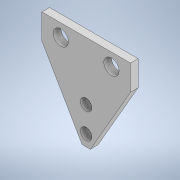
# Autodesk Inventor part: Load Cell Connector to Extrusion Bar
Saved by Autodesk Inventor 2022 (Build 260153000, 153)
## iProperties
Created: 2022-09-20
Part Number: Load Cell Connector to Extrusion Bar
Material: Generic
Document SubType Name: Modeling
Designer: Garrett Raker
Density: 1 g/cm^3
Appearance: Default
Author: Garrett Raker
Autodesk Inventor part; units mm, degrees
ref_plane "YZ Plane" through (0, 0, 0) normal (1, 0, 0) x (0, 1, 0)
ref_plane "XZ Plane" through (0, 0, 0) normal (0, 1, 0) x (-1, 0, 0)
ref_plane "XY Plane" through (0, 0, 0) normal (0, 0, 1) x (1, 0, 0)
sketch "Sketch1" plane through (0, 0, 0) normal (0, 0, 1) x (1, 0, 0)
  circle A0 centre (-10, 13.9812) radius 3
  circle A1 centre (10, 13.9812) radius 3
  circle A2 centre (0, -4.0188) radius 2.25
  circle A3 centre (0, -14.0188) radius 2.25
  line L0 (-1.6291, -18.508) -> (1.6291, -18.508)
  line L1 (-17.5, 8.9812) -> (-1.6291, -18.508)
  line L2 (-17.5, 8.9812) -> (17.1989, 8.9812) construction
  line L3 (17.5, 8.9812) -> (1.6291, -18.508)
  line L4 (17.5, 8.9812) -> (62.1106, 8.9812) construction
  line L5 (-17.5, 8.9812) -> (-17.5, 18.9812)
  line L6 (-17.5, 18.9812) -> (17.5, 18.9812)
  line L7 (17.5, 18.9812) -> (17.5, 8.9812)
  point P0 (0, -18.508)
  dimension "d1" = 4.5
  dimension "d2" = 10
  dimension "d3" = 6
  dimension "d4" = 10
  dimension "d5" = 60
  dimension "d10" = 35
  dimension "d11" = 17.5
  dimension "d13" = 3.2582
  dimension "d17" = 120
  dimension "d20" = 10
  dimension "d22" = 23
  dimension "d26" = 5
  constraints: 16 end point, 5 horizontal, 4 centre point, 2 equal radius, 1 horizontal alignment, 1 midpoint, 1 parallel, 1 perpendicular, 1 vertical, 1 vertical alignment
  measures "d1" diameter of A2
  measures "d2" distance of A2.centre A3.centre
  measures "d3" diameter of A0
  measures "d4" horizontal distance of A1.centre A2.centre
  measures "d5" angle of L1 L2
  measures "d10" distance between parallel lines of L7 L5
  measures "d11" distance from line of A2.centre L5
  measures "d13" distance of L0.start L0.end
  measures "d17" angle of L0 L3
  measures "d20" distance of L1.start L5.end
  measures "d22" distance from line of A2.centre L6
  measures "d26" distance from line of A0.centre L6
extrude "Extrusion1" add sketch "Sketch1" along normal blind 3
ref_plane "Work Plane4" through (-10, 13.9812, 0) normal (1, 0, 0) x (0, 0, -1)
ref_plane "Work Plane1" through (-13, 13.9812, 0) normal (-1, 0, 0) x (0, 0, 1)
ref_plane "Work Plane3" through (-7, 13.9812, 0) normal (1, 0, 0) x (0, 0, -1)
pattern_of_nothing "Mirror1"
ref_plane "Work Plane10" through (-10, 16.9812, 0) normal (0, 1, 0) x (1, 0, 0)
ref_plane "Work Plane12" through (-10, 14.4812, 0) normal (0, 1, 0) x (1, 0, 0)
ref_plane "Work Plane11" through (-10, 11.9812, 0) normal (0, 1, 0) x (1, 0, 0)
ref_plane "Work Plane5" through (10, 13.9812, 0) normal (1, 0, 0) x (0, 0, -1)
equation "\"d11\" = 0.5 * d10"
body "Solid1"
